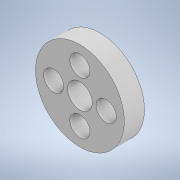
# Autodesk Inventor part: passive_walking_robot6_parts2
Saved by Autodesk Inventor 2021 (Build 250183000, 183)
## iProperties
Created: 2024-06-18
Part Number: passive_walking_robot6_parts2
Material: 一般
Document SubType Name: Modeling
Designer: 山下　響
Density: 1 g/cm^3
Appearance: 既定
Author: 山下　響
Autodesk Inventor part; units mm, degrees
ref_plane "YZ Plane" through (0, 0, 0) normal (1, 0, 0) x (0, 1, 0)
ref_plane "XZ Plane" through (0, 0, 0) normal (0, 1, 0) x (-1, 0, 0)
ref_plane "XY Plane" through (0, 0, 0) normal (0, 0, 1) x (1, 0, 0)
sketch "スケッチ1" plane through (0, 0, 0) normal (0, 0, 1) x (1, 0, 0)
  circle A0 centre (0, 0) radius 3.05
  circle A1 centre (0, 0) radius 11
  circle A2 centre (0, 0) radius 6.5
  circle A3 centre (0, 6.5) radius 2.5
  circle A4 centre (0, -6.5) radius 2.5
  circle A5 centre (6.5, 0) radius 2.5
  circle A6 centre (-6.5, 0) radius 2.5
  dimension "d0" = 6.1
  dimension "d1" = 22
  dimension "d2" = 13
  dimension "d3" = 5
  dimension "d4" = 5
  dimension "d5" = 5
  dimension "d6" = 5
  constraints: 7 centre point, 4 point on circle, 3 coincident
  measures "d0" diameter of A0
  measures "d1" diameter of A1
  measures "d2" diameter of A2
  measures "d3" diameter of A3
  measures "d4" diameter of A4
  measures "d5" diameter of A5
  measures "d6" diameter of A6
extrude "押し出し1" add sketch "スケッチ1" along normal blind 5 contours A1 | A5 A2 A4 A6 A3
